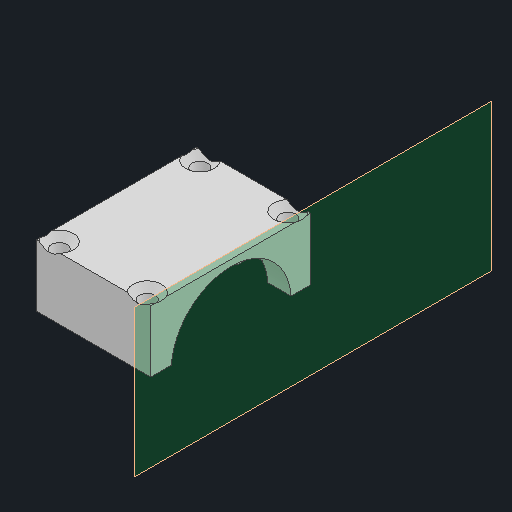
# Autodesk Inventor part: right_motor_ceil
Saved by Autodesk Inventor 2023 (Build 270158000, 158)
## iProperties
Created: 2024-04-14
Part Number: right_motor_ceil
Material: Generic
Document SubType Name: Modeling
Designer: szymo
Density: 1 g/cm^3
Appearance: Default
Author: szymo
Autodesk Inventor part; units mm, degrees
ref_plane "YZ Plane" through (0, 0, 0) normal (1, 0, 0) x (0, 1, 0)
ref_plane "XZ Plane" through (0, 0, 0) normal (0, 1, 0) x (-1, 0, 0)
ref_plane "Work Plane1" through (44.4579, -56.5766, -83.6387) normal (-1, 0, 0) x (0, 0, 1)
sketch "Sketch1" plane through (44.4579, -56.5766, -83.6387) normal (-1, 0, 0) x (0, 0, 1)
  line L0 (90.4615, 0) -> (90.4615, 14.375) projected
  line L1 (90.4615, 14.375) -> (94.9615, 14.375) projected
  arc A0 (94.9615, 14.375) -> (122.2885, 14.375) centre (108.625, 15.375) ccw projected
  line L2 (122.2885, 14.375) -> (127, 14.375) projected
  line L3 (127, 14.375) -> (127, 30.5) projected
  line L4 (52.8275, 30.5) -> (127, 30.5) projected
  line L5 (52.8275, 30.5) -> (52.8275, 10) projected
  line L6 (52.8275, 10) -> (59.8275, 10) projected
  line L7 (59.8275, 10) -> (59.8275, 0) projected
  line L8 (59.8275, 0) -> (90.4615, 0) projected
  line L9 (119.625, 13.875) -> (120.125, 13.875) projected
  line L10 (120.125, 13.875) -> (120.125, 16.875) projected
  line L11 (120.125, 16.875) -> (119.625, 16.875) projected
  line L12 (119.625, 16.875) -> (119.625, 13.875) projected
  line L13 (97.125, 16.875) -> (96.625, 16.875) projected
  line L14 (96.625, 16.875) -> (96.625, 13.875) projected
  line L15 (96.625, 13.875) -> (97.125, 13.875) projected
  line L16 (97.125, 13.875) -> (97.125, 16.875) projected
  circle A1 centre (108.625, 15.375) radius 5 projected
  circle A2 centre (108.625, 15.375) radius 13.7 projected
  line L17 (90.4615, 14.375) -> (127, 14.375)
  line L18 (127, 14.375) -> (127, 30.5)
  line L19 (127, 30.5) -> (90.4615, 30.5)
  line L20 (90.4615, 30.5) -> (90.4615, 14.375)
  line L21 (90.4615, 16.375) -> (127, 16.375)
  point P0 (83.6387, 56.5766)
  point P1 (94.9615, 16.375)
  point P2 (122.2885, 16.375)
  point P3 (127, 16.375)
  dimension "d0" = 2
  constraints: 10 end point, 2 horizontal, 2 parallel, 2 point on line, 1 perpendicular
  measures "d0" distance from line of L21 L0.end
ref_plane "Work Plane2" through (18.3579, -55.5766, 10.6113) normal (1, 0, 0) x (0, 1, 0)
extrude "Extrusion1" add sketch "Sketch1" along normal up to surface (26.1 mm away) contours L20 L4 L3 L21 A2
sketch "Sketch2" plane through (44.4579, -26.0766, 43.3613) normal (0, 1, 0) x (1, 0, 0)
  line L0 (-26.1, 0) -> (-26.1, 4.7115) projected
  line L1 (0, 0) -> (-26.1, 0) projected
  line L2 (0, 4.7115) -> (0, 0) projected
  line L3 (0, 4.7115) -> (-26.1, 4.7115) projected
  line L4 (-26.1, 32.0385) -> (-26.1, 36.5385) projected
  line L5 (0, 32.0385) -> (-26.1, 32.0385) projected
  line L6 (0, 36.5385) -> (0, 32.0385) projected
  line L7 (0, 36.5385) -> (-26.1, 36.5385) projected
  line L8 (-3, 34.3385) -> (-23.1, 34.3385)
  line L9 (-23.1, 34.3385) -> (-23.1, 2.2)
  line L10 (-23.1, 2.2) -> (-3, 2.2)
  line L11 (-3, 2.2) -> (-3, 34.3385)
  point P0 (-44.4579, 43.3613)
  dimension "d3" = 2.2
  dimension "d4" = 2.2
  dimension "d5" = 3
  dimension "d6" = 3
  constraints: 8 end point, 4 coincident, 2 parallel, 1 horizontal, 1 perpendicular
  measures "d3" distance between parallel lines of L7 L8
  measures "d4" distance between parallel lines of L10 L1
  measures "d5" distance between parallel lines of L2 L11
  measures "d6" distance between parallel lines of L4 L9
hole "Hole1" at (41.4579, -26.0766, 9.0229) at (41.4579, -26.0766, 41.1613) at (21.3579, -26.0766, 41.1613) at (21.3579, -26.0766, 9.0229) direction (0, -1, 0) diameter 3.6 end through all countersink diameter 6.5 countersink angle 90
sketch "Sketch3" plane through (44.4579, -40.2016, 6.8229) normal (0, 0, -1) x (-1, 0, 0)
  line L0 (0, 14.125) -> (0.6078, 14.125) projected
  line L1 (0, 14.125) -> (0, 0) projected
  line L2 (0, 0) -> (26.1, 0) projected
  line L3 (26.1, 14.125) -> (26.1, 0) projected
  line L4 (25.4922, 14.125) -> (26.1, 14.125) projected
  line L5 (5.3922, 14.125) -> (20.7078, 14.125) projected
  line L6 (12.3, 0.5) -> (12.3, -2.5) projected
  line L7 (12.3, 0.5) -> (6.3, 0.5) projected
  line L8 (6.3, -2.5) -> (6.3, 0.5) projected
  line L9 (12.3, -2.5) -> (6.3, -2.5) projected
  line L10 (12.3, -14.7) -> (12.3, 12.7) projected
  line L11 (26.1, -2) -> (26.1, -16.375) projected
  line L12 (23.1, -2) -> (26.1, -2) projected
  line L13 (3, -2) -> (23.1, -2) projected
  line L14 (0, -2) -> (3, -2) projected
  line L15 (0, -16.375) -> (0, -2) projected
  line L16 (0, -16.375) -> (26.1, -16.375) projected
  line L17 (12.3, -2) -> (5.3, -2)
  line L18 (5.3, -2) -> (5.3, 5)
  line L19 (5.3, 5) -> (12.3, 5)
  line L20 (12.3, 5) -> (12.3, -2)
  point P0 (44.4579, 40.2016)
  point P1 (12.3, 5)
  point P2 (5.3, -2)
  dimension "d14" = 7
  dimension "d15" = 7
  constraints: 8 end point, 2 horizontal alignment, 2 parallel, 2 point on line, 1 horizontal, 1 perpendicular
  measures "d14" distance of L18.end L19.end
  measures "d15" distance of L17.end L18.end
extrude "Extrusion2" cut sketch "Sketch3" against normal blind 10 contours L18 L19 L10 L7 L8 L2 | L2 L8 L13 L18 | L8 L7 L6 L2 | L2 L6 L13 L8
body "Solid1"
